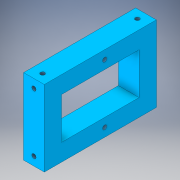
# Autodesk Inventor part: LidarV4Mount
Saved by Autodesk Inventor 2019 (Build 230136000, 136)
## iProperties
Created: 2020-08-15
Part Number: LidarV4Mount
Material: Generic
Document SubType Name: Modeling
Designer: james
Density: 1 g/cm^3
Appearance: Default(1)
Author: james
Autodesk Inventor part; units mm, degrees
ref_plane "YZ Plane" through (0, 0, 0) normal (1, 0, 0) x (0, 1, 0)
ref_plane "XZ Plane" through (0, 0, 0) normal (0, 1, 0) x (-1, 0, 0)
ref_plane "XY Plane" through (0, 0, 0) normal (0, 0, 1) x (1, 0, 0)
sketch "Sketch1" plane through (0, 0, 0) normal (1, 0, 0) x (0, 1, 0)
  line L0 (23.4698, 23.9871) -> (-20.5302, 23.9871)
  line L1 (-20.5302, 23.9871) -> (-20.5302, -41.0129)
  line L2 (-20.5302, -41.0129) -> (23.4698, -41.0129)
  line L3 (23.4698, -41.0129) -> (23.4698, 23.9871)
  point P0 (0, 0)
  dimension "d0" = 44
  dimension "d1" = 65
  constraints: 8 end point, 2 parallel, 1 horizontal, 1 perpendicular
  measures "d0" distance of L1.end L2.end
  measures "d1" distance of L2.end L0.start
extrude "Extrusion1" add sketch "Sketch1" along normal blind 12
sketch "Sketch2" plane through (12, 0, 0) normal (1, 0, 0) x (0, 0, -1)
  line L0 (-13.9871, 13.4698) -> (31.0129, 13.4698)
  line L1 (31.0129, 13.4698) -> (31.0129, -10.5602)
  line L2 (31.0129, -10.5602) -> (-13.9871, -10.5602)
  line L3 (-13.9871, -10.5602) -> (-13.9871, 13.4698)
  line L4 (41.0129, 23.4698) -> (-23.9871, 23.4698) projected
  line L5 (-23.9871, 23.4698) -> (-23.9871, -20.5302) projected
  point P0 (0, 0)
  dimension "d4" = 24.03
  dimension "d5" = 10
  dimension "d6" = 10
  dimension "d7" = 45
  constraints: 8 end point, 2 parallel, 1 horizontal, 1 perpendicular
  measures "d4" distance of L0.end L1.end
  measures "d5" distance between parallel lines of L4 L0
  measures "d6" distance between parallel lines of L5 L3
  measures "d7" distance of L1.end L2.end
extrude "Extrusion2" cut sketch "Sketch2" against normal blind 50.1
sketch "Sketch3" plane through (12, 0, 0) normal (1, 0, 0) x (0, 0, -1)
  line L0 (-23.9871, -20.5302) -> (41.0129, -20.5302) projected
  line L1 (41.0129, 23.4698) -> (-23.9871, 23.4698) projected
  line L2 (41.0129, -20.5302) -> (41.0129, 23.4698) projected
  point P0 (0, 0)
  point P1 (11.0129, 18.4698)
  point P2 (11.0129, -15.5302)
  dimension "d10" = 0
  dimension "d11" = 5
  dimension "d12" = 5
  dimension "d13" = 30
  measures "d10" horizontal distance of point (11.013, -15.53) point (11.013, 18.47)
  measures "d11" distance from line of L0 point (11.013, -15.53)
  measures "d12" distance from line of L1 point (11.013, 18.47)
  measures "d13" distance from line of L2 point (11.013, 18.47)
hole "Hole1" at (12, 18.4698, -11.0129) at (12, -15.5302, -11.0129) direction (-1, 0, 0) diameter 2.4638 end through all
sketch "Sketch4" plane through (0, 23.4698, 23.9871) normal (0, 1, 0) x (1, 0, 0)
  line L0 (0, 0) -> (12, 0) projected
  line L1 (0, 65) -> (12, 65) projected
  line L2 (0, 65) -> (0, 0) projected
  point P0 (0, 23.9871)
  point P1 (6, 5)
  point P2 (6, 60)
  dimension "d21" = 0
  dimension "d22" = 5
  dimension "d23" = 5
  dimension "d24" = 6
  measures "d21" horizontal distance of point (6, 5) point (6, 60)
  measures "d22" distance from line of L0 point (6, 5)
  measures "d23" distance from line of L1 point (6, 60)
  measures "d24" distance from line of L2 point (6, 60)
hole "Hole2" at (6, 23.4698, 18.9871) at (6, 23.4698, -36.0129) direction (0, -1, 0) diameter 2.4638 end through all
sketch "Sketch5" plane through (0, -20.5302, 23.9871) normal (0, 0, 1) x (1, 0, 0)
  line L0 (0, 44) -> (12, 44) projected
  line L1 (0, 0) -> (12, 0) projected
  line L2 (0, 44) -> (0, 0) projected
  point P0 (0, 20.5302)
  point P1 (6, 5)
  point P2 (6, 39)
  dimension "d32" = 0
  dimension "d33" = 5
  dimension "d34" = 5
  dimension "d35" = 6
  measures "d32" horizontal distance of point (6, 39) point (6, 5)
  measures "d33" distance from line of L0 point (6, 39)
  measures "d34" distance from line of L1 point (6, 5)
  measures "d35" distance from line of L2 point (6, 5)
hole "Hole3" at (6, -15.5302, 23.9871) at (6, 18.4698, 23.9871) direction (0, 0, -1) diameter 2.4638 end through all
body "Solid1"
